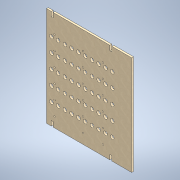
# Autodesk Inventor part: Platte1
Saved by Autodesk Inventor 2020 (Build 240168000, 168)
## iProperties
Created: 2022-03-24
Part Number: Platte1
Material: Pappel
Document SubType Name: Modeling
Designer: Eric
Density: 0.448 g/cm^3
Appearance: Pappel
Author: Eric
Autodesk Inventor part; units mm, degrees
ref_plane "YZ Plane" through (0, 0, 0) normal (1, 0, 0) x (0, 1, 0)
ref_plane "XZ Plane" through (0, 0, 0) normal (0, 1, 0) x (-1, 0, 0)
ref_plane "XY Plane" through (0, 0, 0) normal (0, 0, 1) x (1, 0, 0)
sketch "Skizze1" plane through (0, 0, 0) normal (0, 0, 1) x (1, 0, 0)
  line L0 (0, 0) -> (-180, 0)
  line L1 (-180, 0) -> (-180, 190)
  line L2 (-180, 190) -> (0, 190)
  line L3 (0, 190) -> (0, 0)
  circle A0 centre (-163, 161) radius 1.5
  line L4 (-163, 161) -> (-60.86, 161) construction
  line L5 (-163, 161) -> (-163, 11) construction
  circle A1 centre (-102.72, 161) radius 1.5
  circle A2 centre (-60.86, 161) radius 1.5
  circle A3 centre (-163, 11) radius 1.5
  circle A4 centre (-163, 131) radius 1.5
  circle A5 centre (-163, 101) radius 1.5
  circle A6 centre (-163, 71) radius 1.5
  circle A7 centre (-163, 41) radius 1.5
  circle A8 centre (-102.72, 131) radius 1.5
  circle A9 centre (-102.72, 101) radius 1.5
  circle A10 centre (-102.72, 71) radius 1.5
  circle A11 centre (-102.72, 41) radius 1.5
  circle A12 centre (-102.72, 11) radius 1.5
  circle A13 centre (-60.86, 131) radius 1.5
  circle A14 centre (-60.86, 101) radius 1.5
  circle A15 centre (-60.86, 71) radius 1.5
  circle A16 centre (-60.86, 41) radius 1.5
  circle A17 centre (-60.86, 11) radius 1.5
  dimension "d0" = 180
  dimension "d1" = 190
  dimension "d14" = 60.28
  dimension "d15" = 41.86
  dimension "d16" = 30
  dimension "d17" = 30
  dimension "d18" = 30
  dimension "d19" = 30
  dimension "d20" = 30
  dimension "d21" = 3
  dimension "d22" = 17
  dimension "d23" = 29
  constraints: 18 centre point, 17 equal radius, 12 end point, 10 horizontal alignment, 10 vertical alignment, 5 point on line, 3 coincident, 2 horizontal, 2 parallel, 1 perpendicular, 1 vertical
  measures "d0" distance of L0.start L0.end
  measures "d1" distance of L2.end L0.start
  measures "d14" distance of L4.start A1.centre
  measures "d15" distance of L4.end A1.centre
  measures "d16" distance of A4.centre L4.start
  measures "d17" distance of A5.centre A4.centre
  measures "d18" distance of A6.centre A5.centre
  measures "d19" distance of A7.centre A6.centre
  measures "d20" distance of L5.end A7.centre
  measures "d21" diameter of A0
  measures "d22" distance from line of L1 L4.start
  measures "d23" distance from line of L2 L4.start
extrude "Extrusion1" add sketch "Skizze1" along normal blind 4
sketch "Skizze2" plane through (0, 0, 0) normal (0, 0, -1) x (-1, 0, 0)
  circle A0 centre (41, 4) radius 4
  line L0 (180, 0) -> (0, 0) projected
  line L1 (0, 0) -> (0, 190) projected
  line L2 (41, 4) -> (41, 143) construction
  line L3 (41, 4) -> (133, 4) construction
  circle A1 centre (41, 34) radius 4
  circle A2 centre (41, 64) radius 4
  circle A3 centre (41, 94) radius 4
  circle A4 centre (41, 124) radius 4
  circle A5 centre (55.3, 4) radius 4
  circle A6 centre (55.3, 34) radius 4
  circle A7 centre (55.3, 64) radius 4
  circle A8 centre (55.3, 94) radius 4
  circle A9 centre (55.3, 124) radius 4
  circle A10 centre (69.6, 4) radius 4
  circle A11 centre (69.6, 34) radius 4
  circle A12 centre (69.6, 64) radius 4
  circle A13 centre (69.6, 94) radius 4
  circle A14 centre (69.6, 124) radius 4
  circle A15 centre (83.9, 4) radius 4
  circle A16 centre (83.9, 34) radius 4
  circle A17 centre (83.9, 64) radius 4
  circle A18 centre (83.9, 94) radius 4
  circle A19 centre (83.9, 124) radius 4
  circle A20 centre (98.2, 4) radius 4
  circle A21 centre (98.2, 34) radius 4
  circle A22 centre (98.2, 64) radius 4
  circle A23 centre (98.2, 94) radius 4
  circle A24 centre (98.2, 124) radius 4
  circle A25 centre (112.5, 4) radius 4
  circle A26 centre (112.5, 34) radius 4
  circle A27 centre (112.5, 64) radius 4
  circle A28 centre (112.5, 94) radius 4
  circle A29 centre (112.5, 124) radius 4
  circle A30 centre (126.8, 4) radius 4
  circle A31 centre (126.8, 34) radius 4
  circle A32 centre (126.8, 64) radius 4
  circle A33 centre (126.8, 94) radius 4
  circle A34 centre (126.8, 124) radius 4
  circle A35 centre (141.1, 4) radius 4
  circle A36 centre (141.1, 34) radius 4
  circle A37 centre (141.1, 64) radius 4
  circle A38 centre (141.1, 94) radius 4
  circle A39 centre (141.1, 124) radius 4
  circle A40 centre (155.4, 4) radius 4
  circle A41 centre (155.4, 34) radius 4
  circle A42 centre (155.4, 64) radius 4
  circle A43 centre (155.4, 94) radius 4
  circle A44 centre (155.4, 124) radius 4
  circle A45 centre (169.7, 4) radius 4
  circle A46 centre (169.7, 34) radius 4
  circle A47 centre (169.7, 64) radius 4
  circle A48 centre (169.7, 94) radius 4
  circle A49 centre (169.7, 124) radius 4
  circle A50 centre (41, 154) radius 4
  circle A51 centre (55.3, 154) radius 4
  circle A52 centre (69.6, 154) radius 4
  circle A53 centre (83.9, 154) radius 4
  circle A54 centre (98.2, 154) radius 4
  circle A55 centre (112.5, 154) radius 4
  circle A56 centre (126.8, 154) radius 4
  circle A57 centre (141.1, 154) radius 4
  circle A58 centre (155.4, 154) radius 4
  circle A59 centre (169.7, 154) radius 4
  circle A60 centre (41, 184) radius 4
  circle A61 centre (55.3, 184) radius 4
  circle A62 centre (69.6, 184) radius 4
  circle A63 centre (83.9, 184) radius 4
  circle A64 centre (98.2, 184) radius 4
  circle A65 centre (112.5, 184) radius 4
  circle A66 centre (126.8, 184) radius 4
  circle A67 centre (141.1, 184) radius 4
  circle A68 centre (155.4, 184) radius 4
  circle A69 centre (169.7, 184) radius 4
  dimension "d24" = 8
  dimension "d25" = 4
  dimension "d26" = 41
  dimension "d29" = 30
  dimension "d32" = 14.3
  constraints: 70 centre point, 4 end point, 2 horizontal, 2 vertical, 138 other
  measures "d24" diameter of A0
  measures "d25" distance from line of L0 L2.start
  measures "d26" distance from line of L1 L2.start
  measures "d29" distance of L2.start A1.centre
  measures "d32" distance of L2.start A5.centre
extrude "Extrusion2" cut sketch "Skizze2" against normal blind 4 contours A5 | A10 | A15 | A20 | A25 | A30 | A35 | A40 | A1 | A2 | A3 | A4 | A6 | A7 | A8 | A9 | A11 | A12 | A13 | A14 | A16 | A17 | A18 | A19 | A21 | A22 | A23 | A24 | A26 | A27 | A28 | A29 | A31 | A32 | A33 | A34 | A36 | A37 | A38 | A39 | A41 | A42 | A43 | A44 | A46 | A47 | A48 | A49 | A50 | A51 | A52 | A53 | A54 | A55 | A56 | A57 | A58 | A59 | A61 | A62 | A63 | A64 | A65 | A66 | A67 | A68
sketch "Skizze3" plane through (0, 0, 0) normal (0, 0, -1) x (-1, 0, 0)
  line L0 (180, 190) -> (180, 0) projected
  line L1 (180, 0) -> (180, -10)
  line L2 (180, -10) -> (170, -10)
  line L3 (170, -10) -> (170, 0)
  line L4 (180, 0) -> (0, 0) projected
  line L5 (180, 0) -> (170, 0)
  line L6 (166, 0) -> (46, 0)
  line L7 (46, 0) -> (46, -10)
  line L8 (46, -10) -> (166, -10)
  line L9 (166, -10) -> (166, 0)
  line L10 (0, 0) -> (0, 190) projected
  line L11 (0, 0) -> (42, 0)
  line L12 (42, 0) -> (42, -10)
  line L13 (42, -10) -> (0, -10)
  line L14 (0, -10) -> (0, 0)
  line L15 (0, 190) -> (42, 190)
  line L16 (42, 190) -> (42, 200)
  line L17 (42, 200) -> (0, 200)
  line L18 (0, 200) -> (0, 190)
  line L19 (0, 190) -> (180, 190) projected
  line L20 (46, 190) -> (166, 190)
  line L21 (166, 190) -> (166, 200)
  line L22 (166, 200) -> (46, 200)
  line L23 (46, 200) -> (46, 190)
  line L24 (180, 190) -> (170, 190)
  line L25 (170, 190) -> (170, 200)
  line L26 (170, 200) -> (180, 200)
  line L27 (180, 200) -> (180, 190)
  dimension "d37" = 4
  dimension "d38" = 4
  dimension "d39" = 10
  dimension "d40" = 120
  dimension "d41" = 10
  constraints: 48 end point, 10 parallel, 9 collinear, 7 perpendicular, 5 horizontal, 4 point on line, 1 vertical
  measures "d37" distance between parallel lines of L7 L12
  measures "d38" distance between parallel lines of L9 L3
  measures "d39" distance of L1.end L2.end
  measures "d40" distance between parallel lines of L9 L7
  measures "d41" distance of L0.end L1.end
extrude "Extrusion3" add sketch "Skizze3" against normal blind 4 contours L19 L25 L26 L27 | L1 L2 L3 L4 | L19 L23 L22 L21 | L9 L8 L7 L4 | L15 L18 L17 L16 | L12 L13 L14 L4
equation "\"d17\" = d16"
equation "\"d18\" = d16"
equation "\"d19\" = d16"
equation "\"d20\" = d16"
equation "\"d38\" = d37"
